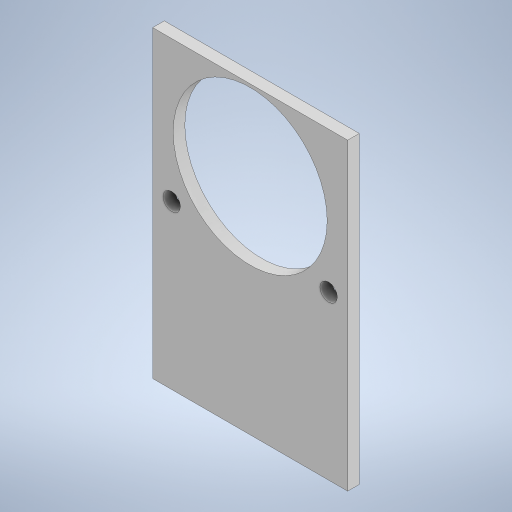
# Autodesk Inventor part: Motor_Cover_2
Saved by Autodesk Inventor 2023.5 (Build 275446020, 446B)
## iProperties
Created: 2025-04-14
Part Number: Motor_Cover_2
Material: Generic
Document SubType Name: Modeling
Designer: Lucky Sah
Density: 1 g/cm^3
Appearance: Default
Author: Lucky Sah
Autodesk Inventor part; units mm, degrees
ref_plane "YZ Plane" through (0, 0, 0) normal (1, 0, 0) x (0, 1, 0)
ref_plane "XZ Plane" through (0, 0, 0) normal (0, 1, 0) x (-1, 0, 0)
ref_plane "XY Plane" through (0, 0, 0) normal (0, 0, 1) x (1, 0, 0)
sketch "Sketch2" plane through (0, 0, 0) normal (0, 0, 1) x (1, 0, 0)
  circle A0 centre (-42.2678, 29.4289) radius 13.25
  line L0 (-25.4928, 43.2039) -> (-59.0428, 43.2039)
  line L1 (-25.4928, -9.0961) -> (-25.4928, 43.2039)
  line L2 (-59.0428, 43.2039) -> (-59.0428, -9.0961)
  line L3 (-59.0428, -9.0961) -> (-25.4928, -9.0961)
  line L4 (-25.4928, -9.0961) -> (-25.4928, 43.2039)
  line L5 (-59.0428, -9.0961) -> (-25.4928, -9.0961)
  circle A1 centre (-55.7678, 18.9289) radius 1.5
  circle A2 centre (-28.7678, 18.9289) radius 1.5
  point P0 (0, 0)
  point P1 (-25.4928, -10.1461)
  dimension "d10" = 26.5
  dimension "d11" = 13.775
  dimension "d12" = 16.775
  dimension "d14" = 3
  dimension "d15" = 10.5
  dimension "d16" = 3
  dimension "d17" = 27
  dimension "d18" = 10.5
  dimension "d19" = 3.275
  dimension "d22" = 52.3
  constraints: 12 end point, 3 centre point, 1 horizontal, 1 perpendicular
  measures "d10" diameter of A0
  measures "d11" distance from line of L0 A0.centre
  measures "d12" distance from line of L1 A0.centre
  measures "d14" diameter of A1
  measures "d15" vertical distance of A1.centre A0.centre
  measures "d16" diameter of A2
  measures "d17" distance of A2.centre A1.centre
  measures "d18" vertical distance of A2.centre A0.centre
  measures "d19" distance from line of L2 A1.centre
  measures "d22" distance between parallel lines of L3 L0
extrude "Extrusion1" add sketch "Sketch2" along normal blind 2
body "Solid1"
